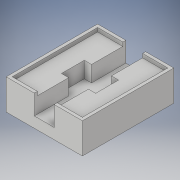
# Autodesk Inventor part: Enclosure_Bottom
Saved by Autodesk Inventor 2017 (Build 210142000, 142)
## iProperties
Created: 2017-11-29
Part Number: Enclosure_Bottom
Material: Generic
Document SubType Name: Modeling
Designer: Tripl_000
Density: 1 g/cm^3
Appearance: Default
Author: Tripl_000
Autodesk Inventor part; units mm, degrees
ref_plane "YZ Plane" through (0, 0, 0) normal (1, 0, 0) x (0, 1, 0)
ref_plane "XZ Plane" through (0, 0, 0) normal (0, 1, 0) x (-1, 0, 0)
ref_plane "XY Plane" through (0, 0, 0) normal (0, 0, 1) x (1, 0, 0)
sketch "Sketch1" plane through (0, 0, 0) normal (0, 1, 0) x (-1, 0, 0)
  line L0 (-25, 30) -> (25, 30)
  line L1 (25, 30) -> (25, -30)
  line L2 (25, -30) -> (-25, -30)
  line L3 (-25, -30) -> (-25, 30)
  line L4 (-25, 30) -> (25, -30) construction
  line L5 (25, 30) -> (-25, -30) construction
  point P0 (0, 0)
  dimension "d0" = 50
  dimension "d1" = 60
  constraints: 12 end point, 2 midpoint, 2 parallel, 1 horizontal, 1 perpendicular
  measures "d0" distance of L1.end L2.end
  measures "d1" distance of L0.end L1.end
extrude "Extrusion1" add sketch "Sketch1" along normal blind 20
sketch "Sketch2" plane through (-25, 0, 30) normal (0, 0, 1) x (1, 0, 0)
  line L0 (0, 20) -> (50, 20) projected
  line L1 (18.5, 20) -> (31.5, 20)
  line L2 (31.5, 20) -> (31.5, 7)
  line L3 (31.5, 7) -> (18.5, 7)
  line L4 (18.5, 7) -> (18.5, 20)
  line L5 (0, 0) -> (0, 20) projected
  point P0 (25, 0)
  dimension "d4" = 13
  dimension "d5" = 13
  dimension "d6" = 18.5
  constraints: 8 end point, 2 parallel, 1 horizontal, 1 perpendicular, 1 point on line
  measures "d4" distance between parallel lines of L2 L4
  measures "d5" distance between parallel lines of L0 L3
  measures "d6" distance between parallel lines of L4 L5
sketch "Sketch3" plane through (0, 20, 0) normal (0, 1, 0) x (1, 0, 0)
  line L0 (-11.25, 7.5) -> (11.25, 7.5)
  line L1 (11.25, 7.5) -> (11.25, -7.5)
  line L2 (11.25, -7.5) -> (-11.25, -7.5)
  line L3 (-11.25, -7.5) -> (-11.25, 7.5)
  line L4 (-11.25, 7.5) -> (11.25, -7.5) construction
  line L5 (11.25, 7.5) -> (-11.25, -7.5) construction
  point P0 (0, 0)
  dimension "d7" = 22.5
  dimension "d8" = 15
  constraints: 12 end point, 2 midpoint, 2 parallel, 1 horizontal, 1 perpendicular
  measures "d7" distance of L0.start L0.end
  measures "d8" distance between parallel lines of L2 L0
shell "Shell1" thickness 2 removed faces 1 at (-8.3333, 20, -10)
sketch "Sketch4" plane through (-23, 2, 28) normal (0, 1, 0) x (1, 0, 0)
  line L0 (0, 0) -> (0, 56) projected
  line L1 (46, 56) -> (46, 0) projected
  line L2 (0, 56) -> (46, 56)
  line L3 (46, 56) -> (46, 0)
  line L4 (46, 0) -> (0, 0)
  line L5 (0, 0) -> (0, 56)
  point P0 (23, 28)
  constraints: 8 end point, 2 parallel, 1 horizontal, 1 perpendicular
extrude "Extrusion2" add sketch "Sketch4" along normal blind 15.5
extrude "Extrusion3" cut sketch "Sketch3" against normal blind 13
extrude "Extrusion4" cut sketch "Sketch2" against normal through all
body "Solid1"
